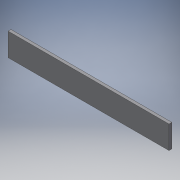
# Autodesk Inventor part: Spoiler
Saved by Autodesk Inventor 2019 (Build 230136000, 136)
## iProperties
Created: 2018-11-27
Part Number: Spoiler
Material: Generic
Document SubType Name: Modeling
Designer: Andres
Density: 1 g/cm^3
Appearance: Default
Author: Andres
Autodesk Inventor part; units mm, degrees
ref_plane "YZ Plane" through (0, 0, 0) normal (1, 0, 0) x (0, 1, 0)
ref_plane "XZ Plane" through (0, 0, 0) normal (0, 1, 0) x (-1, 0, 0)
ref_plane "XY Plane" through (0, 0, 0) normal (0, 0, 1) x (1, 0, 0)
sketch "Sketch1" plane through (0, 0, 0) normal (0, 0, 1) x (1, 0, 0)
  line L0 (3, -4) -> (-53, -4)
  line L1 (-53, -4) -> (-53, 4)
  line L2 (-53, 4) -> (3, 4)
  line L3 (3, 4) -> (3, -4)
  circle A0 centre (0, 0) radius 1.5 projected
  point P0 (0, 0)
  point P1 (-53, 3)
  dimension "d0" = 8
  dimension "d1" = 56
  dimension "d2" = 4
  constraints: 8 end point, 2 parallel, 1 horizontal, 1 perpendicular, 1 other
  measures "d0" distance of L0.end L1.end
  measures "d1" distance of L0.start L0.end
  measures "d2" distance from line of L0 point (0, 0)
extrude "Extrusion2" add sketch "Sketch1" along normal blind 1
body "Solid2"
